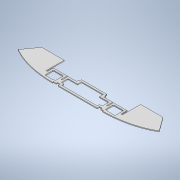
# Autodesk Inventor part: bulkhead_main
Saved by Autodesk Inventor 2022 (Build 260153000, 153)
## iProperties
Created: 2021-04-24
Part Number: bulkhead_main
Material: Generic
Document SubType Name: Modeling
Designer: kardo
Density: 1 g/cm^3
Appearance: Default
Mass: 15.0442 g
Surface Area: 175.344 cm^2
Volume: 15.0442 cm^3
Author: kardo
Autodesk Inventor part; units mm, degrees
ref_plane "YZ Plane" through (0, 0, 0) normal (1, 0, 0) x (0, 1, 0)
ref_plane "XZ Plane" through (0, 0, 0) normal (0, 1, 0) x (-1, 0, 0)
ref_plane "XY Plane" through (0, 0, 0) normal (0, 0, 1) x (1, 0, 0)
derived "frame_outline.ipt"
sketch "bh_main" plane through (0, 0, 0) normal (0, 1, 0) x (-1, 0, 0)
  line L0 (-81, 19.8753) -> (-133.5, 0) construction
  line L1 (-156, 31.008) -> (-133.5, 0) construction
  line L2 (-133.5, 0) -> (-104.625, 0) construction
  line L3 (-81, 4.352) -> (-81, 26.5308) construction
  line L4 (-81, 26.5308) -> (-30, 26.5308) construction
  line L5 (-30, 26.5308) -> (-30, 17.8644) construction
  line L6 (-30, 17.8644) -> (0, 17.8644) construction
  line L7 (-104.625, 0) -> (-81, 0) construction
  line L8 (-81, 4.352) -> (-81, 0) construction
  line L9 (-55, 55.974) -> (0, 55.974) construction
  line L10 (0, 55.174) -> (0, 18.6644)
  line L11 (0, -19.4928) -> (0, 86.9585) construction
  line L12 (0, 55.174) -> (-55, 55.174)
  line L13 (-154.827, 30.7537) -> (-133.0921, 0.8)
  line L14 (-133.0921, 0.8) -> (-81, 0.8)
  line L15 (0, 18.6644) -> (-28, 18.6644)
  line L16 (-28, 18.6644) -> (-28, 27.3308)
  line L17 (-28, 27.3308) -> (-81, 27.3308)
  line L18 (-81, 27.3308) -> (-81, 0.8)
  spline S0 degree 4 poles (-156, 31.008) (-141.197, 39.4592) (-115.7093, 49.7229) (-91.1756, 54.0594) (-64.7341, 55.974) (-55, 55.974) knots 0 0 0 0 0 0.628223 1 1 1 1 1
  spline S1 degree 3 poles (-55, 55.174) (-57.8721, 55.174) (-62.9171, 55.0523) (-68.6715, 54.7173) (-72.9721, 54.3919) (-75.8302, 54.1391) (-79.3894, 53.7801) (-82.2253, 53.4591) (-85.7552, 53.0157) (-88.5673, 52.6269) (-92.7689, 51.9904) (-96.9501, 51.2808) (-102.5023, 50.1987) (-106.6538, 49.2786) (-110.7984, 48.2651) (-113.5582, 47.5419) (-117.0041, 46.5761) (-119.7575, 45.7532) (-123.1946, 44.6603) (-125.9399, 43.734) (-129.3642, 42.5097) (-132.0971, 41.4769) (-135.5019, 40.1186) (-138.2157, 38.9779) (-142.2664, 37.1856) (-147.6278, 34.6514) (-152.2348, 32.2151) (-154.827, 30.7537) knots 0.008263 0.008263 0.008263 0.008263 0.090908 0.152892 0.173553 0.214875 0.235536 0.276859 0.29752 0.338842 0.359503 0.421487 0.462809 0.524793 0.545454 0.586776 0.607438 0.64876 0.669421 0.710743 0.731405 0.772727 0.793388 0.834711 0.855372 0.917355 1 1 1 1
  point P0 (0, 0)
  point P1 (-81, 40.4654)
extrude "Extrusion1" add sketch "bh_main" along normal blind 2
sketch "Sketch2" plane through (0, 2, 55.174) normal (0, 1, 0) x (1, 0, 0)
  line L0 (81, 54.374) -> (81, 27.8432) projected
  line L1 (133.0921, 54.374) -> (81, 54.374) projected
  line L2 (81, 27.8432) -> (81, 14.7086)
  line L3 (81, 14.7086) -> (84, 14.7086)
  line L4 (84, 14.7086) -> (84, 54.374)
  line L5 (81, 27.8432) -> (28, 27.8432) projected
  line L6 (0, 36.5097) -> (0, 0) projected
  point P0 (0, 55.174)
  dimension "d3" = 3
  dimension "d37" = 27.8432
  constraints: 6 end point, 2 point on line, 1 collinear, 1 horizontal, 1 parallel
  measures "d3" distance of L2.end L3.end
  measures "d37" vertical distance of L6.end L0.end
sketch "Sketch3" plane through (0, 2, 55.174) normal (0, 1, 0) x (1, 0, 0)
  line L0 (0, 0) -> (55, 0) projected
  line L1 (55, 0) -> (55, 2)
  line L2 (55, 2) -> (49, 2)
  line L3 (49, 2) -> (49, 5)
  line L4 (49, 5) -> (43, 5)
  line L5 (43, 5) -> (43, 0)
  point P0 (0, 55.174)
  dimension "d6" = 6
  dimension "d7" = 6
  dimension "d8" = 2
  dimension "d9" = 5
  constraints: 10 end point, 3 vertical, 2 horizontal, 1 point on line
  measures "d6" distance of L1.end L2.end
  measures "d7" distance of L3.end L4.end
  measures "d8" distance of L0.end L1.end
  measures "d9" distance of L4.end L5.end
extrude "Extrusion2" cut sketch "Sketch2" against normal through all
extrude "Extrusion3" cut sketch "Sketch3" against normal through all
sketch "Sketch5" plane through (0, 2, 18.6644) normal (0, 1, 0) x (1, 0, 0)
  line L0 (77, -12.6664) -> (77, -31.3553)
  line L1 (77, -31.3553) -> (59, -31.3553)
  line L2 (55, -30.5097) -> (55, -12.6664)
  line L3 (55, -12.6664) -> (77, -12.6664)
  line L4 (81, -21.801) -> (81, -8.6664) projected
  line L5 (81, -8.6664) -> (28, -8.6664) projected
  line L6 (55, -34.5097) -> (55, -36.5097) projected
  line L7 (77, -31.3553) -> (77, -35.3553) construction
  line L8 (59, -31.3553) -> (59, -30.5097)
  line L9 (59, -30.5097) -> (55, -30.5097)
  line L10 (49, -34.5097) -> (55, -34.5097) projected
  line L11 (49, -31.5097) -> (49, -34.5097) projected
  point P0 (0, 18.6644)
  dimension "d21" = 4
  dimension "d22" = 4
  dimension "d24" = 4
  dimension "d42" = 4
  dimension "d43" = 6
  dimension "d44" = 4
  constraints: 14 end point, 6 parallel, 1 collinear, 1 horizontal, 2 other
  measures "d21" distance between parallel lines of L4 L0
  measures "d22" distance between parallel lines of L5 L3
  measures "d24" distance of L0.end L7.end
  measures "d42" distance between parallel lines of L9 L10
  measures "d43" distance between parallel lines of L2 L11
  measures "d44" distance between parallel lines of L6 L8
sketch "Sketch6" plane through (0, 2, 18.6644) normal (0, 1, 0) x (1, 0, 0)
  line L0 (55, -34.5097) -> (55, -36.5097) projected
  line L1 (43, -31.5097) -> (49, -31.5097) projected
  line L2 (43, -36.5097) -> (43, -31.5097) projected
  line L3 (0, -36.5097) -> (43, -36.5097) projected
  line L4 (28, 0) -> (0, 0) projected
  line L5 (28, -8.6664) -> (28, 0) projected
  line L6 (81, -8.6664) -> (28, -8.6664) projected
  line L7 (0, 0) -> (0, -36.5097) projected
  line L8 (0, 0) -> (0, -36.5097) projected
  line L9 (0, -32.5097) -> (39, -32.5097)
  line L10 (39, -32.5097) -> (39, -27.5097)
  line L11 (39, -27.5097) -> (45, -27.5097)
  line L12 (45, -27.5097) -> (45, -12.6664)
  line L13 (45, -12.6664) -> (24, -12.6664)
  line L14 (24, -12.6664) -> (24, -4)
  line L15 (24, -4) -> (0, -4)
  line L16 (49, -31.5097) -> (49, -34.5097) projected
  point P0 (0, 18.6644)
  point P1 (0, -32.5097)
  dimension "d25" = 4
  dimension "d26" = 4
  dimension "d27" = 4
  dimension "d28" = 4
  dimension "d30" = 4
  dimension "d31" = 4
  dimension "d45" = 4
  constraints: 14 end point, 7 parallel, 2 point on line
  measures "d25" distance between parallel lines of L5 L14
  measures "d26" distance between parallel lines of L4 L15
  measures "d27" distance between parallel lines of L3 L9
  measures "d28" distance between parallel lines of L10 L2
  measures "d30" distance between parallel lines of L1 L11
  measures "d31" distance between parallel lines of L6 L13
  measures "d45" distance between parallel lines of L12 L16
extrude "Extrusion5" cut sketch "Sketch5" against normal through all
extrude "Extrusion6" cut sketch "Sketch6" against normal through all
sketch "Sketch7" plane through (0, 2, 18.6644) normal (0, 1, 0) x (1, 0, 0)
  line L0 (81, -8.6664) -> (28, -8.6664) projected
  line L1 (28, -8.6664) -> (28, 0) projected
  line L2 (30, -8.6664) -> (30, -4.3332)
  line L3 (30, -4.3332) -> (28, -4.3332)
  point P0 (0, 18.6644)
  dimension "d39" = 2
  constraints: 4 end point, 2 coincident, 2 parallel, 1 midpoint, 1 point on line, 1 symmetric about line
  measures "d39" distance between parallel lines of L2 L1
extrude "Extrusion7" add sketch "Sketch7" against normal up to surface (2 mm away)
fillet "Fillet1" radius 1.3333 8 edges at (77, 1, 31.3308) (77, 1, 50.0197) (55, 1, 49.174) (55, 1, 31.3308) (45, 1, 31.3308) (45, 1, 46.174) (59, 1, 49.174) (59, 1, 50.0197)
sketch "Sketch9" plane through (0, 2, 18.6644) normal (0, 1, 0) x (1, 0, 0)
  line L0 (81, -8.6664) -> (30, -8.6664) projected
  line L1 (51, -8.6664) -> (51, -21.801)
  line L2 (51, -21.801) -> (49, -21.801)
  line L3 (49, -21.801) -> (49, -8.6664)
  line L4 (84, -21.801) -> (81, -21.801) projected
  line L5 (49, -31.5097) -> (49, -34.5097) projected
  point P0 (0, 18.6644)
  dimension "d47" = 2
  constraints: 6 end point, 2 collinear, 2 point on line, 2 vertical, 1 horizontal
  measures "d47" distance between parallel lines of L3 L1
extrude "Extrusion8" cut sketch "Sketch9" against normal through all
mirror "Mirror1" about plane through (0, 0, 0) normal (1, 0, 0)
equation "\"d1\" = bulkhead_thickness"
equation "\"d3\" = stringer_thickness"
equation "\"d6\" = cowl_liner_width"
equation "\"d7\" = cowl_insulation_width"
equation "\"d8\" = cowl_liner_thickness"
equation "\"d9\" = cowl_liner_thickness + cowl_insulation_thickness"
equation "\"d21\" = inset"
equation "\"d22\" = inset"
equation "\"d24\" = inset"
equation "\"d42\" = inset"
equation "\"d43\" = inset + bulkhead_thickness"
equation "\"d44\" = inset"
equation "\"d25\" = inset"
equation "\"d26\" = inset"
equation "\"d27\" = inset"
equation "\"d28\" = inset"
equation "\"d30\" = inset"
equation "\"d31\" = inset"
equation "\"d45\" = inset"
equation "\"d39\" = bulkhead_thickness"
equation "\"d36\" = 0.333333 * inset"
equation "\"d47\" = bulkhead_thickness"
equation "\"bulkhead_thickness\" = 2"
equation "\"stringer_thickness\" = 3"
equation "\"cowl_liner_width\" = 6"
equation "\"cowl_insulation_width\" = 6"
equation "\"cowl_liner_thickness\" = 2"
equation "\"cowl_insulation_thickness\" = 3"
equation "\"inset\" = 4"
body "Solid1"
